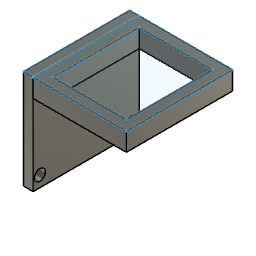
switch mount (Autodesk Fusion 360 design; units mm, degrees)
Autodesk Fusion 360 part; units mm, degrees
sketch "Sketch5" plane through (0, 0, 0) normal (0, 0, 1) x (1, 0, 0)
  line L0 (40, 25) -> (20, 25)
  line L1 (20, 25) -> (20, 1.5)
  line L2 (20, 1.5) -> (40, 1.5)
  line L3 (40, 1.5) -> (40, 25)
  line L4 (42.7186, -1.2186) -> (42.7186, 27.7186)
  line L5 (42.7186, 27.7186) -> (17.2814, 27.7186)
  line L6 (17.2814, 27.7186) -> (17.2814, -1.2186)
  line L7 (17.2814, -1.2186) -> (42.7186, -1.2186)
  line L8 (17.2814, 27.7186) -> (14.6795, 27.7186)
  line L9 (14.6795, 27.7186) -> (14.6795, -1.199)
  line L10 (14.6795, -1.199) -> (17.2814, -1.199)
  line L11 (17.2814, -1.199) -> (17.2814, 27.7186)
  dimension "d10" = 20
  dimension "d11" = 23.5
  dimension "d12" = 2.7186
  constraint horizontal L0
  constraint vertical L1
  constraint horizontal L2
  constraint vertical L3
  constraint horizontal L8
  constraint vertical L9
  constraint horizontal L10
  constraint vertical L11
  measures "d10" distance of L0.start L0.end
  measures "d11" distance of L0.start L2.end
extrude "Extrude4" add sketch "Sketch5" against normal blind 5 contours L4 L5 L6 L7 L11 makes body 1
extrude "Extrude5" add sketch "Sketch5" against normal blind 27 separate body contours L6 L8 L9 L10 L11 makes body 2
sketch "Sketch8" plane through (0, 0, 0) normal (1, 0, 0) x (0, 1, 0)
  circle A0 centre (25.6551, -24) radius 1.5
  circle A1 centre (0.6551, -24) radius 1.5
  dimension "d17" = 3
  dimension "d18" = 25
  dimension "d19" = 3
  measures "d17" diameter of A0
  measures "d18" distance of A0.centre A1.centre
  measures "d19" diameter of A1
sketch "Sketch10" plane through (0, 0, 0) normal (1, 0, 0) x (0, 1, 0)
  line L0 (-1.269, -0.0277, 14.6645) -> (-5.269, -0.0277, 14.6645)
  line L1 (-5.269, -0.0277, 14.6645) -> (-5.269, -27.0277, 14.6645)
  line L2 (-5.269, -27.0277, 14.6645) -> (-1.269, -27.0277, 14.6645)
  line L3 (-1.269, -27.0277, 14.6645) -> (-1.269, -0.0277, 14.6645)
  line L4 (26.731, -0.0277, 14.6645) -> (30.731, -0.0277, 14.6645)
  line L5 (30.731, -0.0277, 14.6645) -> (30.731, -27.0277, 14.6645)
  line L6 (30.731, -27.0277, 14.6645) -> (26.731, -27.0277, 14.6645)
  line L7 (26.731, -27.0277, 14.6645) -> (26.731, -0.0277, 14.6645)
extrude "Extrude6" cut sketch "Sketch8" along normal blind 35 bodies 2
